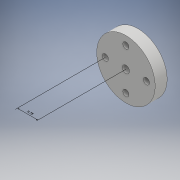
# Autodesk Inventor part: Polonier AX
Saved by Autodesk Inventor 2018 (Build 220112000, 112)
## iProperties
Part Number: Polonier AX
Material: Générique
Document SubType Name: Modeling
Designer: Thomas
Density: 1 g/cm^3
Appearance: Par défaut
Author: Thomas
Autodesk Inventor part; units mm, degrees
ref_plane "YZ Plane" through (0, 0, 0) normal (1, 0, 0) x (0, 1, 0)
ref_plane "XZ Plane" through (0, 0, 0) normal (0, 1, 0) x (-1, 0, 0)
ref_plane "XY Plane" through (0, 0, 0) normal (0, 0, 1) x (1, 0, 0)
sketch "Esquisse1" plane through (0, 0, 0) normal (0, 1, 0) x (-1, 0, 0)
  circle A0 centre (0, 0) radius 11
  line L0 (0, 0) -> (7.75, 0)
  circle A1 centre (7.75, 0) radius 1.15
  line L1 (8.8758, -1.95) -> (6.6242, -1.95)
  line L2 (6.6242, -1.95) -> (5.4983, 0)
  line L3 (5.4983, 0) -> (6.6242, 1.95)
  line L4 (6.6242, 1.95) -> (8.8758, 1.95)
  line L5 (8.8758, 1.95) -> (10.0017, 0)
  line L6 (10.0017, 0) -> (8.8758, -1.95)
  line L7 (0, 0) -> (0, 7.75)
  circle A2 centre (0, 7.75) radius 1.15
  line L8 (1.95, 8.8758) -> (1.95, 6.6242)
  line L9 (1.95, 6.6242) -> (0, 5.4983)
  line L10 (0, 5.4983) -> (-1.95, 6.6242)
  line L11 (-1.95, 6.6242) -> (-1.95, 8.8758)
  line L12 (-1.95, 8.8758) -> (0, 10.0017)
  line L13 (0, 10.0017) -> (1.95, 8.8758)
  line L14 (0, 0) -> (-7.75, 0)
  circle A3 centre (-7.75, 0) radius 1.15
  line L15 (-8.8758, 1.95) -> (-6.6242, 1.95)
  line L16 (-6.6242, 1.95) -> (-5.4983, 0)
  line L17 (-5.4983, 0) -> (-6.6242, -1.95)
  line L18 (-6.6242, -1.95) -> (-8.8758, -1.95)
  line L19 (-8.8758, -1.95) -> (-10.0017, 0)
  line L20 (-10.0017, 0) -> (-8.8758, 1.95)
  line L21 (0, 0) -> (0, -7.75)
  circle A4 centre (0, -7.75) radius 1.15
  line L22 (-1.95, -8.8758) -> (-1.95, -6.6242)
  line L23 (-1.95, -6.6242) -> (0, -5.4983)
  line L24 (0, -5.4983) -> (1.95, -6.6242)
  line L25 (1.95, -6.6242) -> (1.95, -8.8758)
  line L26 (1.95, -8.8758) -> (0, -10.0017)
  line L27 (0, -10.0017) -> (-1.95, -8.8758)
  dimension "d0" = 22
  dimension "d1" = 7.75
  dimension "d2" = 2.3
  dimension "d3" = 3.9
  dimension "d6" = 360
  constraints: 56 end point, 9 coincident, 5 centre point, 1 horizontal, 86 other
  measures "d0" diameter of A0
  measures "d1" distance of L0.start L0.end
  measures "d2" diameter of A1
  measures "d3" distance between parallel lines of L1 L4
extrude "Extrusion1" add sketch "Esquisse1" along normal blind 4.5 contours A0 | L3 L4 L5 L6 L1 L2 | L10 L11 L12 L13 L8 L9 | L17 L18 L19 L20 L15 L16 | L24 L25 L26 L27 L22 L23
sketch "Esquisse2" plane through (0, 4.5, 0) normal (0, 1, 0) x (1, 0, 0)
  circle A0 centre (-7.75, 0) radius 1.15 projected
  line L0 (-10.1171, 0) -> (-8.9336, 2.05)
  line L1 (-8.9336, 2.05) -> (-6.5664, 2.05)
  line L2 (-6.5664, 2.05) -> (-5.3829, 0)
  line L3 (-5.3829, 0) -> (-6.5664, -2.05)
  line L4 (-6.5664, -2.05) -> (-8.9336, -2.05)
  line L5 (-8.9336, -2.05) -> (-10.1171, 0)
  line L6 (-8.9626, 3.15) -> (-5.9313, 3.15)
  line L7 (-5.9313, 3.15) -> (-5.18, 1.8486)
  line L8 (-5.18, -1.8486) -> (-5.9313, -3.15)
  line L9 (-5.9313, -3.15) -> (-8.9626, -3.15)
  arc A1 (-5.4134, 0.0529) -> (-5.4134, -0.0529) centre (0, 0) ccw
  circle A2 centre (0, 0) radius 11 projected
  line L10 (2.05, -6.5664) -> (2.05, -8.9336)
  line L11 (2.05, -8.9336) -> (0, -10.1171)
  line L12 (3.15, -5.9313) -> (3.15, -8.9626)
  arc A3 (-0.0529, -5.4134) -> (0.0529, -5.4134) centre (0, 0) ccw
  line L13 (0, -5.3829) -> (2.05, -6.5664)
  line L14 (1.8486, -5.18) -> (3.15, -5.9313)
  line L15 (0, -10.1171) -> (-2.05, -8.9336)
  line L16 (-2.05, -8.9336) -> (-2.05, -6.5664)
  line L17 (-2.05, -6.5664) -> (0, -5.3829)
  line L18 (-3.15, -8.9626) -> (-3.15, -5.9313)
  line L19 (-3.15, -5.9313) -> (-1.8486, -5.18)
  line L20 (6.5664, 2.05) -> (8.9336, 2.05)
  line L21 (8.9336, 2.05) -> (10.1171, 0)
  line L22 (5.9313, 3.15) -> (8.9626, 3.15)
  arc A4 (5.4134, -0.0529) -> (5.4134, 0.0529) centre (0, 0) ccw
  line L23 (5.3829, 0) -> (6.5664, 2.05)
  line L24 (5.18, 1.8486) -> (5.9313, 3.15)
  line L25 (10.1171, 0) -> (8.9336, -2.05)
  line L26 (8.9336, -2.05) -> (6.5664, -2.05)
  line L27 (6.5664, -2.05) -> (5.3829, 0)
  line L28 (8.9626, -3.15) -> (5.9313, -3.15)
  line L29 (5.9313, -3.15) -> (5.18, -1.8486)
  line L30 (-2.05, 6.5664) -> (-2.05, 8.9336)
  line L31 (-2.05, 8.9336) -> (0, 10.1171)
  line L32 (-3.15, 5.9313) -> (-3.15, 8.9626)
  arc A5 (0.0529, 5.4134) -> (-0.0529, 5.4134) centre (0, 0) ccw
  line L33 (0, 5.3829) -> (-2.05, 6.5664)
  line L34 (-1.8486, 5.18) -> (-3.15, 5.9313)
  line L35 (0, 10.1171) -> (2.05, 8.9336)
  line L36 (2.05, 8.9336) -> (2.05, 6.5664)
  line L37 (2.05, 6.5664) -> (0, 5.3829)
  line L38 (3.15, 8.9626) -> (3.15, 5.9313)
  line L39 (3.15, 5.9313) -> (1.8486, 5.18)
  arc A6 (-8.9626, -3.15) -> (-3.15, -8.9626) centre (0, 0) ccw
  arc A7 (-3.15, 8.9626) -> (-8.9626, 3.15) centre (0, 0) ccw
  arc A8 (3.15, -8.9626) -> (8.9626, -3.15) centre (0, 0) ccw
  arc A9 (8.9626, 3.15) -> (3.15, 8.9626) centre (0, 0) ccw
  arc A10 (5.4134, -0.0529) -> (5.4134, 0.0529) centre (0, 0) ccw
  arc A11 (1.8486, -5.18) -> (5.18, -1.8486) centre (0, 0) ccw
  arc A12 (-5.18, -1.8486) -> (-1.8486, -5.18) centre (0, 0) ccw
  arc A13 (-0.0529, -5.4134) -> (0.0529, -5.4134) centre (0, 0) ccw
  arc A14 (-1.8486, 5.18) -> (-5.18, 1.8486) centre (0, 0) ccw
  arc A15 (5.18, 1.8486) -> (1.8486, 5.18) centre (0, 0) ccw
  arc A16 (0.0529, 5.4134) -> (-0.0529, 5.4134) centre (0, 0) ccw
  arc A17 (-3.15, 8.9098) -> (-8.9098, 3.15) centre (0, 0) ccw
  arc A18 (-8.9098, -3.15) -> (-3.15, -8.9098) centre (0, 0) ccw
  arc A19 (3.15, -8.9098) -> (8.9098, -3.15) centre (0, 0) ccw
  arc A20 (8.9098, 3.15) -> (3.15, 8.9098) centre (0, 0) ccw
  point P0 (0, -7.75)
  point P1 (0, -7.75)
  point P2 (7.75, 0)
  point P3 (7.75, 0)
  point P4 (0, 7.75)
  point P5 (0, 7.75)
  dimension "d10" = 4.1
  dimension "d16" = 360
  constraints: 80 end point, 38 point on circle, 19 centre point, 16 point on line, 6 coincident, 126 other
  measures "d10" distance between parallel lines of L1 L4
extrude "Extrusion2" cut sketch "Esquisse2" against normal blind 2.6 contours L0 L1 L2 A1 L3 L4 L5 | A7 L32 A17 L6 | A17 L32 L34 A14 L7 L6 | A12 L19 L18 A18 L9 L8 | A18 L18 A6 L9 | L10 L11 L15 L16 L17 A3 L13 | L14 A11 L29 L28 A19 L12 | A19 L28 A8 L12 | L20 L21 L25 L26 L27 A4 L23 | L24 A15 L39 L38 A20 L22 | A20 L38 A9 L22 | L30 L31 L35 L36 L37 A5 L33
sketch "Esquisse3" plane through (0, 4.5, 0) normal (0, 1, 0) x (1, 0, 0)
  line L0 (-3.3057, 0) -> (-2.9057, 0) construction
  line L1 (-2.9057, 0) -> (-3.2832, -0.3321)
  line L2 (-2.9057, 0) -> (-3.2832, 0.3321)
  line L3 (-2.788, -0.8186) -> (-3.2438, -0.6064)
  line L4 (-2.788, -0.8186) -> (-3.0567, -1.2436)
  line L5 (-2.4445, -1.571) -> (-2.9416, -1.4957)
  line L6 (-2.4445, -1.571) -> (-2.5825, -2.0544)
  line L7 (-1.9029, -2.196) -> (-2.401, -2.2639)
  line L8 (-1.9029, -2.196) -> (-1.8991, -2.6988)
  line L9 (-1.2071, -2.6432) -> (-1.666, -2.8486)
  line L10 (-1.2071, -2.6432) -> (-1.0618, -3.1245)
  line L11 (-0.4135, -2.8762) -> (-0.796, -3.2026)
  line L12 (-0.4135, -2.8762) -> (-0.1386, -3.2971)
  line L13 (0.4135, -2.8762) -> (0.1386, -3.2971)
  line L14 (0.4135, -2.8762) -> (0.796, -3.2026)
  line L15 (1.2071, -2.6432) -> (1.0618, -3.1245)
  line L16 (1.2071, -2.6432) -> (1.666, -2.8486)
  line L17 (1.9029, -2.196) -> (1.8991, -2.6988)
  line L18 (1.9029, -2.196) -> (2.401, -2.2639)
  line L19 (2.4445, -1.571) -> (2.5825, -2.0544)
  line L20 (2.4445, -1.571) -> (2.9416, -1.4957)
  line L21 (2.788, -0.8186) -> (3.0567, -1.2436)
  line L22 (2.788, -0.8186) -> (3.2438, -0.6064)
  line L23 (2.9057, 0) -> (3.2832, -0.3321)
  line L24 (2.9057, 0) -> (3.2832, 0.3321)
  line L25 (2.788, 0.8186) -> (3.2438, 0.6064)
  line L26 (2.788, 0.8186) -> (3.0567, 1.2436)
  line L27 (2.4445, 1.571) -> (2.9416, 1.4957)
  line L28 (2.4445, 1.571) -> (2.5825, 2.0544)
  line L29 (1.9029, 2.196) -> (2.401, 2.2639)
  line L30 (1.9029, 2.196) -> (1.8991, 2.6988)
  line L31 (1.2071, 2.6432) -> (1.666, 2.8486)
  line L32 (1.2071, 2.6432) -> (1.0618, 3.1245)
  line L33 (0.4135, 2.8762) -> (0.796, 3.2026)
  line L34 (0.4135, 2.8762) -> (0.1386, 3.2971)
  line L35 (-0.4135, 2.8762) -> (-0.1386, 3.2971)
  line L36 (-0.4135, 2.8762) -> (-0.796, 3.2026)
  line L37 (-1.2071, 2.6432) -> (-1.0618, 3.1245)
  line L38 (-1.2071, 2.6432) -> (-1.666, 2.8486)
  line L39 (-1.9029, 2.196) -> (-1.8991, 2.6988)
  line L40 (-1.9029, 2.196) -> (-2.401, 2.2639)
  line L41 (-2.4445, 1.571) -> (-2.5825, 2.0544)
  line L42 (-2.4445, 1.571) -> (-2.9416, 1.4957)
  line L43 (-2.788, 0.8186) -> (-3.0567, 1.2436)
  line L44 (-2.788, 0.8186) -> (-3.2438, 0.6064)
  arc A0 (-3.2438, 0.6064) -> (-3.2832, 0.3321) centre (0, 0) ccw
  arc A1 (-2.9416, 1.4957) -> (-3.0567, 1.2436) centre (0, 0) ccw
  arc A2 (-2.401, 2.2639) -> (-2.5825, 2.0544) centre (0, 0) ccw
  arc A3 (-1.666, 2.8486) -> (-1.8991, 2.6988) centre (0, 0) ccw
  arc A4 (-0.796, 3.2026) -> (-1.0618, 3.1245) centre (0, 0) ccw
  arc A5 (0.1386, 3.2971) -> (-0.1386, 3.2971) centre (0, 0) ccw
  arc A6 (1.0618, 3.1245) -> (0.796, 3.2026) centre (0, 0) ccw
  arc A7 (1.8991, 2.6988) -> (1.666, 2.8486) centre (0, 0) ccw
  arc A8 (2.5825, 2.0544) -> (2.401, 2.2639) centre (0, 0) ccw
  arc A9 (3.0567, 1.2436) -> (2.9416, 1.4957) centre (0, 0) ccw
  arc A10 (3.2832, 0.3321) -> (3.2438, 0.6064) centre (0, 0) ccw
  arc A11 (3.2438, -0.6064) -> (3.2832, -0.3321) centre (0, 0) ccw
  arc A12 (2.9416, -1.4957) -> (3.0567, -1.2436) centre (0, 0) ccw
  arc A13 (2.401, -2.2639) -> (2.5825, -2.0544) centre (0, 0) ccw
  arc A14 (1.666, -2.8486) -> (1.8991, -2.6988) centre (0, 0) ccw
  arc A15 (0.796, -3.2026) -> (1.0618, -3.1245) centre (0, 0) ccw
  arc A16 (-0.1386, -3.2971) -> (0.1386, -3.2971) centre (0, 0) ccw
  arc A17 (-1.0618, -3.1245) -> (-0.796, -3.2026) centre (0, 0) ccw
  arc A18 (-1.8991, -2.6988) -> (-1.666, -2.8486) centre (0, 0) ccw
  arc A19 (-2.5825, -2.0544) -> (-2.401, -2.2639) centre (0, 0) ccw
  arc A20 (-3.2832, -0.3321) -> (-3.2438, -0.6064) centre (0, 0) ccw
  arc A21 (-3.0567, -1.2436) -> (-2.9416, -1.4957) centre (0, 0) ccw
  circle A22 centre (0, 0) radius 4.55
  arc A23 (-3.2438, 0.6064) -> (-3.2438, -0.6064) centre (0, 0) ccw construction
  dimension "d22" = 0.4
  dimension "d25" = 360
  dimension "d40" = 9.1
  dimension "d41" = 3.3
  constraints: 90 end point, 46 point on circle, 24 centre point, 2 coincident, 1 horizontal, 1 symmetric about line, 111 other
  measures "d22" distance of L0.start L0.end
  measures "d40" diameter of A22
  measures "d41" radius of A20
extrude "Extrusion3" add sketch "Esquisse3" along normal blind 2.3
sketch "Esquisse4" plane through (0, 4.5, 0) normal (0, 1, 0) x (1, 0, 0)
  line L0 (-3.2832, 0.3321) -> (-2.9057, 0) projected
  line L1 (-2.9057, 0) -> (-3.2832, -0.3321) projected
  arc A0 (-3.2832, -0.3321) -> (-3.2438, -0.6064) centre (0, 0) ccw projected
  line L2 (-3.2438, -0.6064) -> (-2.788, -0.8186) projected
  line L3 (-2.788, -0.8186) -> (-3.0567, -1.2436) projected
  arc A1 (-3.0567, -1.2436) -> (-2.9416, -1.4957) centre (0, 0) ccw projected
  line L4 (-2.9416, -1.4957) -> (-2.4445, -1.571) projected
  line L5 (-2.4445, -1.571) -> (-2.5825, -2.0544) projected
  arc A2 (-2.5825, -2.0544) -> (-2.401, -2.2639) centre (0, 0) ccw projected
  line L6 (-2.401, -2.2639) -> (-1.9029, -2.196) projected
  line L7 (-1.9029, -2.196) -> (-1.8991, -2.6988) projected
  arc A3 (-1.8991, -2.6988) -> (-1.666, -2.8486) centre (0, 0) ccw projected
  line L8 (-1.666, -2.8486) -> (-1.2071, -2.6432) projected
  line L9 (-1.2071, -2.6432) -> (-1.0618, -3.1245) projected
  arc A4 (-1.0618, -3.1245) -> (-0.796, -3.2026) centre (0, 0) ccw projected
  line L10 (-0.796, -3.2026) -> (-0.4135, -2.8762) projected
  line L11 (-0.4135, -2.8762) -> (-0.1386, -3.2971) projected
  arc A5 (-0.1386, -3.2971) -> (0.1386, -3.2971) centre (0, 0) ccw projected
  line L12 (0.1386, -3.2971) -> (0.4135, -2.8762) projected
  line L13 (0.4135, -2.8762) -> (0.796, -3.2026) projected
  arc A6 (0.796, -3.2026) -> (1.0618, -3.1245) centre (0, 0) ccw projected
  line L14 (1.0618, -3.1245) -> (1.2071, -2.6432) projected
  line L15 (1.2071, -2.6432) -> (1.666, -2.8486) projected
  arc A7 (1.666, -2.8486) -> (1.8991, -2.6988) centre (0, 0) ccw projected
  line L16 (1.8991, -2.6988) -> (1.9029, -2.196) projected
  line L17 (1.9029, -2.196) -> (2.401, -2.2639) projected
  arc A8 (2.401, -2.2639) -> (2.5825, -2.0544) centre (0, 0) ccw projected
  line L18 (2.5825, -2.0544) -> (2.4445, -1.571) projected
  line L19 (2.4445, -1.571) -> (2.9416, -1.4957) projected
  arc A9 (2.9416, -1.4957) -> (3.0567, -1.2436) centre (0, 0) ccw projected
  line L20 (3.0567, -1.2436) -> (2.788, -0.8186) projected
  line L21 (2.788, -0.8186) -> (3.2438, -0.6064) projected
  arc A10 (3.2438, -0.6064) -> (3.2832, -0.3321) centre (0, 0) ccw projected
  line L22 (3.2832, -0.3321) -> (2.9057, 0) projected
  line L23 (2.9057, 0) -> (3.2832, 0.3321) projected
  arc A11 (3.2832, 0.3321) -> (3.2438, 0.6064) centre (0, 0) ccw projected
  line L24 (3.2438, 0.6064) -> (2.788, 0.8186) projected
  line L25 (2.788, 0.8186) -> (3.0567, 1.2436) projected
  arc A12 (3.0567, 1.2436) -> (2.9416, 1.4957) centre (0, 0) ccw projected
  line L26 (2.9416, 1.4957) -> (2.4445, 1.571) projected
  line L27 (2.4445, 1.571) -> (2.5825, 2.0544) projected
  arc A13 (2.5825, 2.0544) -> (2.401, 2.2639) centre (0, 0) ccw projected
  line L28 (2.401, 2.2639) -> (1.9029, 2.196) projected
  line L29 (1.9029, 2.196) -> (1.8991, 2.6988) projected
  arc A14 (1.8991, 2.6988) -> (1.666, 2.8486) centre (0, 0) ccw projected
  line L30 (1.666, 2.8486) -> (1.2071, 2.6432) projected
  line L31 (1.2071, 2.6432) -> (1.0618, 3.1245) projected
  arc A15 (1.0618, 3.1245) -> (0.796, 3.2026) centre (0, 0) ccw projected
  line L32 (0.796, 3.2026) -> (0.4135, 2.8762) projected
  line L33 (0.4135, 2.8762) -> (0.1386, 3.2971) projected
  arc A16 (0.1386, 3.2971) -> (-0.1386, 3.2971) centre (0, 0) ccw projected
  line L34 (-0.1386, 3.2971) -> (-0.4135, 2.8762) projected
  line L35 (-0.4135, 2.8762) -> (-0.796, 3.2026) projected
  arc A17 (-0.796, 3.2026) -> (-1.0618, 3.1245) centre (0, 0) ccw projected
  line L36 (-1.0618, 3.1245) -> (-1.2071, 2.6432) projected
  line L37 (-1.2071, 2.6432) -> (-1.666, 2.8486) projected
  arc A18 (-1.666, 2.8486) -> (-1.8991, 2.6988) centre (0, 0) ccw projected
  line L38 (-1.8991, 2.6988) -> (-1.9029, 2.196) projected
  line L39 (-1.9029, 2.196) -> (-2.401, 2.2639) projected
  arc A19 (-2.401, 2.2639) -> (-2.5825, 2.0544) centre (0, 0) ccw projected
  line L40 (-2.5825, 2.0544) -> (-2.4445, 1.571) projected
  line L41 (-2.4445, 1.571) -> (-2.9416, 1.4957) projected
  arc A20 (-2.9416, 1.4957) -> (-3.0567, 1.2436) centre (0, 0) ccw projected
  line L42 (-3.0567, 1.2436) -> (-2.788, 0.8186) projected
  line L43 (-2.788, 0.8186) -> (-3.2438, 0.6064) projected
  arc A21 (-3.2438, 0.6064) -> (-3.2832, 0.3321) centre (0, 0) ccw projected
extrude "Extrusion4" cut sketch "Esquisse4" against normal blind 2.3
sketch "Esquisse5" plane through (0, 2.2, 0) normal (0, 1, 0) x (1, 0, 0)
  circle A0 centre (0, 0) radius 1.35
  dimension "d31" = 2.7
  constraints: 1 centre point, 1 coincident
  measures "d31" diameter of A0
extrude "Extrusion5" cut sketch "Esquisse5" against normal blind 2.3
